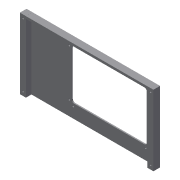
# Autodesk Inventor part: 04_OPENTRONS_Microscope_wellplate_base
Saved by Autodesk Inventor 2019.4 (Build 234330000, 330)
## iProperties
Created: 2020-11-05
Part Number: 04_OPENTRONS_Microscope_wellplate_base
Material: Generic
Document SubType Name: Modeling
Designer: diederichbenedict
Density: 1 g/cm^3
Appearance: Default
Author: diederichbenedict
Autodesk Inventor part; units mm, degrees
ref_plane "YZ Plane" through (0, 0, 0) normal (1, 0, 0) x (0, 1, 0)
ref_plane "XZ Plane" through (0, 0, 0) normal (0, 1, 0) x (-1, 0, 0)
ref_plane "XY Plane" through (0, 0, 0) normal (0, 0, 1) x (1, 0, 0)
sketch "Sketch1" plane through (0, 0, 0) normal (0, 0, 1) x (1, 0, 0)
  line L0 (-133.7, 52.6137) -> (86.8, 52.6137)
  line L1 (86.8, 52.6137) -> (86.8, -63.9)
  line L2 (86.8, -63.9) -> (-133.7, -63.9)
  line L3 (-133.7, -63.9) -> (-133.7, 52.6137)
  line L4 (-149.2, -74.9) -> (-149.2, -103.9) construction
  line L5 (86.8, -114.9) -> (86.8, -63.9) construction
  line L6 (-133.7, 52.7) -> (-133.7, -51.9) projected
  line L7 (-133.7, -63.9) -> (-123.7, -63.9) projected
  line L8 (64.8, 41.6) -> (16.1, 41.6) construction
  arc A0 (68.7, 37.7) -> (64.8, 41.6) centre (64.8, 37.7) ccw construction
  line L9 (68.7, -39.9) -> (68.7, 37.7) construction
  arc A1 (64.8, -43.8) -> (68.7, -39.9) centre (64.8, -39.9) ccw construction
  line L10 (16.1, -43.8) -> (64.8, -43.8) construction
  line L11 (16.1, -42.3) -> (16.1, -43.8) construction
  line L12 (60.6858, -42.3) -> (16.1, -42.3) construction
  arc A2 (60.6858, -42.3) -> (61.4636, -41.9778) centre (60.6858, -41.2) ccw construction
  line L13 (66.8778, -36.5636) -> (61.4636, -41.9778) construction
  arc A3 (66.8778, -36.5636) -> (67.2, -35.7858) centre (66.1, -35.7858) ccw construction
  line L14 (67.2, 33.5858) -> (67.2, -35.7858) construction
  arc A4 (67.2, 33.5858) -> (66.8778, 34.3636) centre (66.1, 33.5858) ccw construction
  line L15 (61.4636, 39.7778) -> (66.8778, 34.3636) construction
  arc A5 (61.4636, 39.7778) -> (60.6858, 40.1) centre (60.6858, 39) ccw construction
  line L16 (16.1, 40.1) -> (60.6858, 40.1) construction
  line L17 (16.1, 41.6) -> (16.1, 40.1) construction
  line L18 (-6.3, 41.6) -> (-55, 41.6) construction
  line L19 (-6.3, 40.1) -> (-6.3, 41.6) construction
  line L20 (-55.3, 40.1) -> (-6.3, 40.1) construction
  arc A6 (-55.3, 40.1) -> (-57.4, 38) centre (-55.3, 38) ccw construction
  line L21 (-57.4, -40.2) -> (-57.4, 38) construction
  arc A7 (-57.4, -40.2) -> (-55.3, -42.3) centre (-55.3, -40.2) ccw construction
  line L22 (-6.3, -42.3) -> (-55.3, -42.3) construction
  line L23 (-6.3, -43.8) -> (-6.3, -42.3) construction
  line L24 (-55, -43.8) -> (-6.3, -43.8) construction
  arc A8 (-58.9, -39.9) -> (-55, -43.8) centre (-55, -39.9) ccw construction
  line L25 (-58.9, 37.7) -> (-58.9, -39.9) construction
  arc A9 (-55, 41.6) -> (-58.9, 37.7) centre (-55, 37.7) ccw construction
  line L26 (62.7, -41.8) -> (-53.4, -41.8)
  line L27 (-57.4, -37.8) -> (-57.4, 35.6)
  line L28 (-53.4, 39.6) -> (62.7, 39.6)
  line L29 (66.7, 35.6) -> (66.7, -37.8)
  arc A10 (-53.4, 39.6) -> (-57.4, 35.6) centre (-53.4, 35.6) ccw
  arc A11 (-57.4, -37.8) -> (-53.4, -41.8) centre (-53.4, -37.8) ccw
  arc A12 (66.7, 35.6) -> (62.7, 39.6) centre (62.7, 35.6) ccw
  arc A13 (62.7, -41.8) -> (66.7, -37.8) centre (62.7, -37.8) ccw
  dimension "d15" = 0
  dimension "d47" = 0
  dimension "d50" = 0
  dimension "d54" = 4
  dimension "d55" = 2
  dimension "d56" = 2
  dimension "d57" = 2
  constraints: 14 end point, 8 point on circle, 8 tangent, 4 centre point, 3 equal radius, 3 parallel, 2 horizontal, 1 perpendicular, 1 vertical, 3 other
  measures "d15" distance between parallel lines of L1 L5
  measures "d47" distance between parallel lines of L6 L3
  measures "d50" distance between parallel lines of L2 L7
  measures "d54" radius of A10
  measures "d55" distance between parallel lines of L28 L18
  measures "d56" distance between parallel lines of L29 L9
  measures "d57" distance between parallel lines of L26 L10
extrude "Extrusion1" add sketch "Sketch1" along normal blind 2
hole "Hole1" at (71, 37.7, 0) at (64.8, 43.9, 0) at (71, -39.9, 0) at (64.8, -46.1, 0) at (-55, -46.3, 0) at (-61.4, -39.9, 0) at (-61.4, 37.7, 0) at (-56.5875, 43.9, 0) direction (0, 0, 1) diameter 2.9 end through all
ref_plane "Work Plane3" through (-133.7, 41.6084, 11.0916) normal (0, 0, -1) x (0, 1, 0)
sketch "Sketch3" plane through (0, 0, 2) normal (0, 0, 1) x (1, 0, 0)
  line L0 (86.8, 52.6137) -> (-133.7, 52.6137) projected
  line L1 (-133.7, 52.6137) -> (-133.7, -63.9) projected
  line L2 (-133.7, -63.9) -> (86.8, -63.9) projected
  line L3 (86.8, -63.9) -> (86.8, 52.6137) projected
  line L4 (86.8, -63.9) -> (86.8, 52.6137) projected
  line L5 (-133.7, 52.6137) -> (-133.7, -63.9) projected
  line L6 (86.8, -63.9) -> (-133.7, -63.9)
  line L7 (-133.7, -63.9) -> (-133.7, -59.9)
  line L8 (-133.7, -59.9) -> (86.8, -59.9)
  line L9 (86.8, -59.9) -> (86.8, -63.9)
  line L10 (-133.7, 52.6137) -> (86.8, 52.6137)
  line L11 (86.8, 52.6137) -> (86.8, 48.6137)
  line L12 (86.8, 48.6137) -> (-133.7, 48.6137)
  line L13 (-133.7, 48.6137) -> (-133.7, 52.6137)
  arc A0 (66.7, 35.6) -> (62.7, 39.6) centre (62.7, 35.6) ccw projected
  line L14 (66.7, 35.6) -> (66.7, -37.8) projected
  arc A1 (62.7, -41.8) -> (66.7, -37.8) centre (62.7, -37.8) ccw projected
  line L15 (62.7, -41.8) -> (-53.4, -41.8) projected
  arc A2 (-57.4, -37.8) -> (-53.4, -41.8) centre (-53.4, -37.8) ccw projected
  line L16 (-57.4, -37.8) -> (-57.4, 35.6) projected
  arc A3 (-53.4, 39.6) -> (-57.4, 35.6) centre (-53.4, 35.6) ccw projected
  line L17 (-53.4, 39.6) -> (62.7, 39.6) projected
  point P0 (0, 0)
  dimension "d17" = 4
  dimension "d18" = 4
  constraints: 16 end point, 4 parallel, 2 horizontal, 2 perpendicular, 2 point on line
  measures "d17" distance of L6.end L7.end
  measures "d18" distance of L10.end L11.end
extrude "Extrusion2" add sketch "Sketch3" along normal up to surface (9.0916 mm away) contours L3 L12 L1 L0
sketch "Sketch8" plane through (0, 0, 2) normal (0, 0, 1) x (1, 0, 0)
  line L0 (-123.7, 52.7) -> (-123.7, -51.9) projected
  circle A0 centre (-128.7, 47.1542) radius 1.45 projected
  line L1 (76.8, 52.7) -> (76.8, -51.9) projected
  line L2 (86.8, -114.9) -> (86.8, 52.7) projected
  line L3 (-133.7, 52.7) -> (-133.7, -51.9) projected
  line L4 (-133.7, 52.7) -> (-123.7, 52.7)
  line L5 (-123.7, 52.7) -> (-123.7, -63.9)
  line L6 (-123.7, -63.9) -> (-133.7, -63.9)
  line L7 (-133.7, -63.9) -> (-133.7, 52.7)
  line L8 (86.8, -63.9) -> (-133.7, -63.9) projected
  line L9 (86.8, 52.7) -> (76.8, 52.7)
  line L10 (76.8, 52.7) -> (76.8, -63.9)
  line L11 (76.8, -63.9) -> (86.8, -63.9)
  line L12 (86.8, -63.9) -> (86.8, 52.7)
  point P0 (0, 0)
  constraints: 16 end point, 4 parallel, 4 point on line, 2 horizontal, 2 perpendicular
ref_plane "Work Plane2" through (-133.7, 41.6084, 11.0916) normal (0, 0, -1) x (0, 1, 0)
extrude "Extrusion5" add sketch "Sketch8" along normal up to surface (9.0916 mm away)
sketch "Sketch9" plane through (0, 0, 0) normal (0, 0, -1) x (-1, 0, 0)
  circle A0 centre (128.7, -57.3542) radius 1.45 projected
  circle A1 centre (128.7, 47.1542) radius 1.45 projected
  circle A2 centre (-81.8, -57.3542) radius 1.45 projected
  circle A3 centre (-81.8, 47.1542) radius 1.45 projected
  point P0 (0, 0)
hole "Hole4" at (81.8, 47.1542, 0) at (81.8, -57.3542, 0) at (-128.7, 47.1542, 0) at (-128.7, -57.3542, 0) direction (0, 0, 1) diameter 4.3 end through all
body "Solid1"
